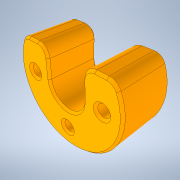
# Autodesk Inventor part: Проставка катушки левая
Saved by Autodesk Inventor 2021.1 (Build 251245010, 245A)
## iProperties
Created: 2026-04-16
Part Number: Проставка катушки левая
Material: Типовые
Document SubType Name: Modeling
Designer: Андрей Тарасов
Density: 1 g/cm^3
Appearance: По умолчанию
Author: Андрей Тарасов
Autodesk Inventor part; units mm, degrees
ref_plane "YZ Plane" through (0, 0, 0) normal (1, 0, 0) x (0, 1, 0)
ref_plane "XZ Plane" through (0, 0, 0) normal (0, 1, 0) x (-1, 0, 0)
ref_plane "XY Plane" through (0, 0, 0) normal (0, 0, 1) x (1, 0, 0)
sketch "Эскиз1" plane through (0, 0, 0) normal (0, 0, 1) x (1, 0, 0)
  circle A0 centre (0, 0) radius 5.1
  circle A1 centre (0, 0) radius 15
  line L0 (0, -21) -> (0, 21) construction
  line L1 (-21, 0) -> (21, 0) construction
  circle A2 centre (0, 0) radius 10.05 construction
  circle A3 centre (-10.05, 0) radius 1.6
  circle A4 centre (0, -10.05) radius 1.6
  circle A5 centre (10.05, 0) radius 1.6
  line L2 (-12.6886, 8) -> (12.6886, 8)
  line L3 (-5.1, 0) -> (-5.1, 8)
  line L4 (5.1, 0) -> (5.1, 8)
  dimension "d0" = 10.2
  dimension "d1" = 30
  dimension "d2" = 20.1
  dimension "d3" = 3.2
  dimension "d4" = 8
  constraints: 7 point on circle, 6 centre point, 6 end point, 6 point on line, 3 coincident, 2 equal radius, 2 perpendicular, 2 tangent, 1 horizontal
  measures "d0" diameter of A0
  measures "d1" diameter of A1
  measures "d2" diameter of A2
  measures "d3" diameter of A5
  measures "d4" distance between parallel lines of L2 L1
extrude "Выдавливание1" add sketch "Эскиз1" along normal blind 14 contours L4 L2 A1 L3 A0
fillet "Сопряжение1" radius 3 4 edges at (-12.6886, 8, 7) (-5.1, 8, 7) (5.1, 8, 7) (12.6886, 8, 7)
chamfer "Фаска1" distance 0.6 angle 45 26 edges at (-5.9787, 7.1213, 14) (-5.1, 2.5, 14) (0, -5.1, 14) (5.1, 2.5, 14) (5.9787, 7.1213, 14) (9.5044, 8, 14) (12.5289, 7.5249, 14) (0, -15, 14) (-12.5289, 7.5249, 14) (-9.5044, 8, 14) (-11.65, 0, 14) (-1.6, -10.05, 14) (8.45, 0, 14) (0, -5.1, 0) (-5.1, 2.5, 0) (-5.9787, 7.1213, 0) (-9.5044, 8, 0) (-12.5289, 7.5249, 0) (0, -15, 0) (12.5289, 7.5249, 0) (9.5044, 8, 0) (5.9787, 7.1213, 0) (5.1, 2.5, 0) (-11.65, 0, 0) (-1.6, -10.05, 0) (8.45, 0, 0)
equation "\"d2\" = 0.5 * d0 + 0.5 * d1"
